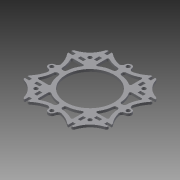
# Autodesk Inventor part: Plate2
Saved by Autodesk Inventor 2014 SP1 (Build 180222100, 222)
## iProperties
Created: 2014-07-27
Part Number: Plate2
Material: Generic
Document SubType Name: Modeling
Designer: Ryan
Density: 1 g/cm^3
Appearance: Default
Author: Ryan
Autodesk Inventor part; units mm, degrees
ref_plane "YZ Plane" through (0, 0, 0) normal (1, 0, 0) x (0, 1, 0)
ref_plane "XZ Plane" through (0, 0, 0) normal (0, 1, 0) x (-1, 0, 0)
ref_plane "XY Plane" through (0, 0, 0) normal (0, 0, 1) x (1, 0, 0)
sketch "Plate2" plane through (0, 0, 0) normal (0, 0, 1) x (1, 0, 0)
  arc A0 (128.4552, 70.0073) -> (126.9175, 69.5516) centre (128.2368, 67.9221) ccw
  arc A1 (95.9929, 69.5516) -> (94.4552, 70.0073) centre (94.6736, 67.9221) ccw
  arc A2 (85.5189, 60.9436) -> (90.0883, 68.5842) centre (72.6151, 73.8474) ccw
  arc A3 (92.0552, 69.9919) -> (90.0883, 68.5842) centre (91.9751, 68.0259) ccw
  arc A4 (132.8221, 68.5842) -> (137.3915, 60.9436) centre (150.2953, 73.8474) ccw
  arc A5 (132.8221, 68.5842) -> (130.8552, 69.9919) centre (130.9353, 68.0259) ccw
  circle A6 centre (111.4552, 35.0073) radius 20
  line L0 (94.4552, 70.0073) -> (94.4552, 66.3006)
  line L1 (92.0552, 69.9919) -> (92.0552, 66.3006)
  line L2 (92.0552, 66.3006) -> (94.4552, 66.3006)
  line L3 (130.8552, 69.9919) -> (130.8552, 66.3073)
  line L4 (128.4552, 70.0073) -> (128.4552, 66.3073)
  line L5 (128.4552, 66.3073) -> (130.8552, 66.3073)
  line L6 (96.8417, 55.1789) -> (96.8417, 63.4787)
  arc A7 (98.3161, 64.359) -> (108.0321, 61.6397) centre (109.2141, 84.5799) ccw
  arc A8 (98.3161, 64.359) -> (96.8417, 63.4787) centre (97.8417, 63.4787) ccw
  arc A9 (109.4549, 60.1414) -> (108.0321, 61.6397) centre (107.9549, 60.1417) ccw
  arc A10 (108.0698, 57.6324) -> (98.3885, 54.3416) centre (109.6496, 37.0981) ccw
  arc A11 (96.8417, 55.1789) -> (98.3885, 54.3416) centre (97.8417, 55.1789) ccw
  arc A12 (108.0698, 57.6324) -> (109.4548, 59.1277) centre (107.9548, 59.128) ccw
  line L7 (109.4548, 59.1277) -> (109.4549, 60.1414)
  line L8 (126.0687, 55.1789) -> (126.0687, 63.4787)
  arc A13 (114.8782, 61.6397) -> (124.5943, 64.359) centre (113.6962, 84.5799) ccw
  arc A14 (126.0687, 63.4787) -> (124.5943, 64.359) centre (125.0687, 63.4787) ccw
  arc A15 (114.8782, 61.6397) -> (113.4554, 60.1414) centre (114.9554, 60.1417) ccw
  arc A16 (124.5219, 54.3416) -> (114.8405, 57.6324) centre (113.2608, 37.0981) ccw
  arc A17 (124.5219, 54.3416) -> (126.0687, 55.1789) centre (125.0687, 55.1789) ccw
  arc A18 (113.4556, 59.1277) -> (114.8405, 57.6324) centre (114.9556, 59.128) ccw
  line L9 (113.4556, 59.1277) -> (113.4554, 60.1414)
  line L10 (131.6268, 49.6208) -> (139.9266, 49.6208)
  arc A19 (140.8069, 48.1464) -> (138.0875, 38.4304) centre (161.0277, 37.2484) ccw
  arc A20 (140.8069, 48.1464) -> (139.9266, 49.6208) centre (139.9266, 48.6208) ccw
  arc A21 (136.5893, 37.0076) -> (138.0875, 38.4304) centre (136.5895, 38.5076) ccw
  arc A22 (134.0802, 38.3927) -> (130.7895, 48.074) centre (113.5459, 36.8129) ccw
  arc A23 (131.6268, 49.6208) -> (130.7895, 48.074) centre (131.6268, 48.6208) ccw
  arc A24 (134.0802, 38.3927) -> (135.5756, 37.0077) centre (135.5758, 38.5077) ccw
  line L11 (135.5756, 37.0077) -> (136.5893, 37.0076)
  line L12 (91.2836, 49.6208) -> (82.9838, 49.6208)
  arc A25 (84.8228, 38.4304) -> (82.1035, 48.1464) centre (61.8827, 37.2484) ccw
  arc A26 (82.9838, 49.6208) -> (82.1035, 48.1464) centre (82.9838, 48.6208) ccw
  arc A27 (84.8228, 38.4304) -> (86.3211, 37.0076) centre (86.3208, 38.5076) ccw
  arc A28 (92.1209, 48.074) -> (88.8301, 38.3927) centre (109.3644, 36.8129) ccw
  arc A29 (92.1209, 48.074) -> (91.2836, 49.6208) centre (91.2836, 48.6208) ccw
  arc A30 (87.3348, 37.0077) -> (88.8301, 38.3927) centre (87.3345, 38.5077) ccw
  line L13 (87.3348, 37.0077) -> (86.3211, 37.0076)
  arc A31 (145.9995, 50.4696) -> (146.4552, 52.0073) centre (144.3699, 51.7889) ccw
  arc A32 (137.3915, 60.9436) -> (145.032, 56.3742) centre (150.2953, 73.8474) ccw
  arc A33 (146.4397, 54.4073) -> (145.032, 56.3742) centre (144.4737, 54.4874) ccw
  line L14 (146.4397, 54.4073) -> (142.7552, 54.4073)
  line L15 (146.4552, 52.0073) -> (142.7552, 52.0073)
  line L16 (142.7552, 52.0073) -> (142.7552, 54.4073)
  arc A34 (81.7248, 40.9245) -> (76.9109, 50.4696) centre (58.1218, 35.0073) ccw
  arc A35 (76.4552, 52.0073) -> (76.9109, 50.4696) centre (78.5404, 51.7889) ccw
  arc A36 (77.8783, 56.3742) -> (85.5189, 60.9436) centre (72.6151, 73.8474) ccw
  arc A37 (77.8783, 56.3742) -> (76.4706, 54.4073) centre (78.4366, 54.4874) ccw
  line L17 (76.4552, 52.0073) -> (80.1619, 52.0073)
  line L18 (76.4706, 54.4073) -> (80.1619, 54.4073)
  line L19 (80.1619, 54.4073) -> (80.1619, 52.0073)
  arc A38 (126.9175, 0.463) -> (128.4552, 0.0073) centre (128.2368, 2.0926) ccw
  arc A39 (94.4552, 0.0073) -> (95.9929, 0.463) centre (94.6736, 2.0926) ccw
  arc A40 (90.0883, 1.4305) -> (85.5189, 9.071) centre (72.6151, -3.8328) ccw
  arc A41 (90.0883, 1.4305) -> (92.0552, 0.0228) centre (91.9751, 1.9888) ccw
  arc A42 (137.3915, 9.071) -> (132.8221, 1.4305) centre (150.2953, -3.8328) ccw
  arc A43 (130.8552, 0.0228) -> (132.8221, 1.4305) centre (130.9353, 1.9888) ccw
  line L20 (94.4552, 0.0073) -> (94.4552, 3.7141)
  line L21 (92.0552, 0.0228) -> (92.0552, 3.7141)
  line L22 (92.0552, 3.7141) -> (94.4552, 3.7141)
  line L23 (130.8552, 0.0228) -> (130.8552, 3.7073)
  line L24 (128.4552, 0.0073) -> (128.4552, 3.7073)
  line L25 (128.4552, 3.7073) -> (130.8552, 3.7073)
  line L26 (96.8417, 14.8357) -> (96.8417, 6.5359)
  arc A44 (108.0321, 8.375) -> (98.3161, 5.6556) centre (109.2141, -14.5652) ccw
  arc A45 (96.8417, 6.5359) -> (98.3161, 5.6556) centre (97.8417, 6.5359) ccw
  arc A46 (108.0321, 8.375) -> (109.4549, 9.8732) centre (107.9549, 9.873) ccw
  arc A47 (98.3885, 15.673) -> (108.0698, 12.3823) centre (109.6496, 32.9166) ccw
  arc A48 (98.3885, 15.673) -> (96.8417, 14.8357) centre (97.8417, 14.8357) ccw
  arc A49 (109.4548, 10.8869) -> (108.0698, 12.3823) centre (107.9548, 10.8867) ccw
  line L27 (109.4548, 10.8869) -> (109.4549, 9.8732)
  line L28 (126.0687, 14.8357) -> (126.0687, 6.5359)
  arc A50 (124.5943, 5.6556) -> (114.8782, 8.375) centre (113.6962, -14.5652) ccw
  arc A51 (124.5943, 5.6556) -> (126.0687, 6.5359) centre (125.0687, 6.5359) ccw
  arc A52 (113.4554, 9.8732) -> (114.8782, 8.375) centre (114.9554, 9.873) ccw
  arc A53 (114.8405, 12.3823) -> (124.5219, 15.673) centre (113.2608, 32.9166) ccw
  arc A54 (126.0687, 14.8357) -> (124.5219, 15.673) centre (125.0687, 14.8357) ccw
  arc A55 (114.8405, 12.3823) -> (113.4556, 10.8869) centre (114.9556, 10.8867) ccw
  line L29 (113.4556, 10.8869) -> (113.4554, 9.8732)
  line L30 (131.6268, 20.3938) -> (139.9266, 20.3938)
  arc A56 (138.0875, 31.5843) -> (140.8069, 21.8682) centre (161.0277, 32.7663) ccw
  arc A57 (139.9266, 20.3938) -> (140.8069, 21.8682) centre (139.9266, 21.3938) ccw
  arc A58 (138.0875, 31.5843) -> (136.5893, 33.0071) centre (136.5895, 31.5071) ccw
  arc A59 (130.7895, 21.9406) -> (134.0802, 31.622) centre (113.5459, 33.2017) ccw
  arc A60 (130.7895, 21.9406) -> (131.6268, 20.3938) centre (131.6268, 21.3938) ccw
  arc A61 (135.5756, 33.0069) -> (134.0802, 31.622) centre (135.5758, 31.5069) ccw
  line L31 (135.5756, 33.0069) -> (136.5893, 33.0071)
  line L32 (91.2836, 20.3938) -> (82.9838, 20.3938)
  arc A62 (82.1035, 21.8682) -> (84.8228, 31.5843) centre (61.8827, 32.7663) ccw
  arc A63 (82.1035, 21.8682) -> (82.9838, 20.3938) centre (82.9838, 21.3938) ccw
  arc A64 (86.3211, 33.0071) -> (84.8228, 31.5843) centre (86.3208, 31.5071) ccw
  arc A65 (88.8301, 31.622) -> (92.1209, 21.9406) centre (109.3644, 33.2017) ccw
  arc A66 (91.2836, 20.3938) -> (92.1209, 21.9406) centre (91.2836, 21.3938) ccw
  arc A67 (88.8301, 31.622) -> (87.3348, 33.0069) centre (87.3345, 31.5069) ccw
  line L33 (87.3348, 33.0069) -> (86.3211, 33.0071)
  arc A68 (146.4552, 18.0073) -> (145.9995, 19.545) centre (144.3699, 18.2257) ccw
  arc A69 (145.032, 13.6404) -> (137.3915, 9.071) centre (150.2953, -3.8328) ccw
  arc A70 (145.032, 13.6404) -> (146.4397, 15.6073) centre (144.4737, 15.5272) ccw
  line L34 (146.4397, 15.6073) -> (142.7552, 15.6073)
  line L35 (146.4552, 18.0073) -> (142.7552, 18.0073)
  line L36 (142.7552, 18.0073) -> (142.7552, 15.6073)
  arc A71 (76.9109, 19.545) -> (81.7248, 29.0902) centre (58.1218, 35.0073) ccw
  arc A72 (76.9109, 19.545) -> (76.4552, 18.0073) centre (78.5404, 18.2257) ccw
  arc A73 (85.5189, 9.071) -> (77.8783, 13.6404) centre (72.6151, -3.8328) ccw
  arc A74 (76.4706, 15.6073) -> (77.8783, 13.6404) centre (78.4366, 15.5272) ccw
  line L37 (76.4552, 18.0073) -> (80.1619, 18.0073)
  line L38 (76.4706, 15.6073) -> (80.1619, 15.6073)
  line L39 (80.1619, 15.6073) -> (80.1619, 18.0073)
  circle A75 centre (79.6354, 35.0073) radius 1.6
  circle A76 centre (88.9552, 12.5073) radius 1.6
  circle A77 centre (88.9552, 57.5073) radius 1.6
  circle A78 centre (133.9552, 57.5073) radius 1.6
  circle A79 centre (133.9552, 12.5073) radius 1.6
  arc A80 (76.8156, 35.0073) -> (79.4575, 32.1931) centre (79.6354, 35.0073) ccw
  arc A81 (79.4575, 37.8215) -> (76.8156, 35.0073) centre (79.6354, 35.0073) ccw
  arc A82 (79.4575, 37.8215) -> (81.7248, 40.9245) centre (79.2998, 40.3165) ccw
  arc A83 (81.7248, 29.0902) -> (79.4575, 32.1931) centre (79.2998, 29.6981) ccw
  arc A84 (95.9929, 69.5516) -> (105.538, 64.7377) centre (111.4552, 88.3407) ccw
  arc A85 (117.3723, 64.7377) -> (126.9175, 69.5516) centre (111.4552, 88.3407) ccw
  arc A86 (114.2694, 67.005) -> (117.3723, 64.7377) centre (116.7644, 67.1627) ccw
  circle A87 centre (111.4552, 66.8271) radius 1.6
  arc A88 (114.2694, 67.005) -> (111.4552, 69.6469) centre (111.4552, 66.8271) ccw
  arc A89 (111.4552, 69.6469) -> (108.641, 67.005) centre (111.4552, 66.8271) ccw
  arc A90 (105.538, 64.7377) -> (108.641, 67.005) centre (106.146, 67.1627) ccw
  arc A91 (145.9995, 50.4696) -> (141.1856, 40.9245) centre (164.7885, 35.0073) ccw
  arc A92 (141.1856, 29.0902) -> (145.9995, 19.545) centre (164.7885, 35.0073) ccw
  arc A93 (143.4528, 32.1931) -> (141.1856, 29.0902) centre (143.6105, 29.6981) ccw
  circle A94 centre (143.275, 35.0073) radius 1.6
  arc A95 (143.4528, 32.1931) -> (146.0948, 35.0073) centre (143.275, 35.0073) ccw
  arc A96 (146.0948, 35.0073) -> (143.4528, 37.8215) centre (143.275, 35.0073) ccw
  arc A97 (141.1856, 40.9245) -> (143.4528, 37.8215) centre (143.6105, 40.3165) ccw
  arc A98 (105.538, 5.2769) -> (95.9929, 0.463) centre (111.4552, -18.326) ccw
  arc A99 (126.9175, 0.463) -> (117.3723, 5.2769) centre (111.4552, -18.326) ccw
  arc A100 (117.3723, 5.2769) -> (114.2694, 3.0097) centre (116.7644, 2.852) ccw
  circle A101 centre (111.4552, 3.1875) radius 1.6
  arc A102 (111.4552, 0.3677) -> (114.2694, 3.0097) centre (111.4552, 3.1875) ccw
  arc A103 (108.641, 3.0097) -> (111.4552, 0.3677) centre (111.4552, 3.1875) ccw
  arc A104 (108.641, 3.0097) -> (105.538, 5.2769) centre (106.146, 2.852) ccw
  line L40 (84.3552, 52.0073) -> (84.3552, 54.4073)
  line L41 (84.3552, 54.4073) -> (88.7552, 54.4073)
  line L42 (88.7552, 54.4073) -> (88.7552, 52.0073)
  line L43 (88.7552, 52.0073) -> (84.3552, 52.0073)
  line L44 (138.5552, 54.4073) -> (134.1552, 54.4073)
  line L45 (134.1552, 54.4073) -> (134.1552, 52.0072)
  line L46 (134.1552, 52.0072) -> (138.5552, 52.0073)
  line L47 (138.5552, 52.0073) -> (138.5552, 54.4073)
  line L48 (84.3552, 18.0073) -> (84.3552, 15.6073)
  line L49 (84.3552, 15.6073) -> (88.7552, 15.6073)
  line L50 (84.3552, 18.0073) -> (88.7552, 18.0073)
  line L51 (88.7552, 18.0073) -> (88.7552, 15.6073)
  line L52 (138.5552, 18.0073) -> (138.5552, 15.6073)
  line L53 (138.5552, 15.6073) -> (134.1552, 15.6073)
  line L54 (138.5552, 18.0073) -> (134.1552, 18.0073)
  line L55 (134.1552, 18.0073) -> (134.1552, 15.6073)
  line L56 (92.0552, 62.1073) -> (94.4552, 62.1073)
  line L57 (94.4552, 62.1073) -> (94.4552, 57.7073)
  line L58 (92.0552, 62.1073) -> (92.0552, 57.7073)
  line L59 (92.0552, 57.7073) -> (94.4552, 57.7073)
  line L60 (128.4552, 62.1073) -> (130.8552, 62.1073)
  line L61 (130.8552, 62.1073) -> (130.8552, 57.7073)
  line L62 (128.4552, 62.1073) -> (128.4552, 57.7073)
  line L63 (128.4552, 57.7073) -> (130.8552, 57.7073)
  line L64 (128.4552, 7.9073) -> (130.8552, 7.9073)
  line L65 (130.8552, 7.9073) -> (130.8552, 12.3073)
  line L66 (128.4552, 7.9073) -> (128.4552, 12.3073)
  line L67 (128.4552, 12.3073) -> (130.8552, 12.3073)
  line L68 (92.0552, 7.9073) -> (94.4552, 7.9073)
  line L69 (94.4552, 7.9073) -> (94.4552, 12.3073)
  line L70 (92.0552, 7.9073) -> (92.0552, 12.3073)
  line L71 (92.0552, 12.3073) -> (94.4552, 12.3073)
  point P0 (111.4553, 35.0073)
sketch "Sketch1" plane through (0, 0, 0) normal (0, 1, 0) x (-1, 0, 0)
  circle A0 centre (35.6381, 35.0073) radius 20
  circle A1 centre (67.4579, 35.0073) radius 1.6
  circle A2 centre (35.6381, 66.8271) radius 1.6
  circle A3 centre (13.1381, 57.5073) radius 1.6
  circle A4 centre (58.1381, 57.5073) radius 1.6
  circle A5 centre (3.8183, 35.0073) radius 1.6
  circle A6 centre (13.1381, 12.5073) radius 1.6
  circle A7 centre (35.6381, 3.1875) radius 1.6
  circle A8 centre (58.1381, 12.5073) radius 1.6
  line L0 (8.5381, 54.4073) -> (12.9381, 54.4073)
  line L1 (12.9381, 54.4073) -> (12.9381, 52.0073)
  line L2 (12.9381, 52.0073) -> (8.5381, 52.0073)
  line L3 (8.5381, 52.0073) -> (8.5381, 54.4073)
  line L4 (16.2381, 62.1073) -> (18.6381, 62.1073)
  line L5 (18.6381, 62.1073) -> (18.6381, 57.7073)
  line L6 (18.6381, 57.7073) -> (16.2381, 57.7073)
  line L7 (16.2381, 57.7073) -> (16.2381, 62.1073)
  line L8 (52.6381, 62.1073) -> (55.0381, 62.1073)
  line L9 (55.0381, 62.1073) -> (55.0381, 57.7073)
  line L10 (55.0381, 57.7073) -> (52.6381, 57.7073)
  line L11 (52.6381, 57.7073) -> (52.6381, 62.1073)
  line L12 (58.3381, 54.4073) -> (62.7381, 54.4073)
  line L13 (62.7381, 54.4073) -> (62.7381, 52.0073)
  line L14 (62.7381, 52.0073) -> (58.3381, 52.0073)
  line L15 (58.3381, 52.0073) -> (58.3381, 54.4073)
  line L16 (58.3381, 18.0073) -> (62.7381, 18.0073)
  line L17 (62.7381, 18.0073) -> (62.7381, 15.6073)
  line L18 (62.7381, 15.6073) -> (58.3381, 15.6073)
  line L19 (58.3381, 15.6073) -> (58.3381, 18.0073)
  line L20 (52.6381, 12.3073) -> (55.0381, 12.3073)
  line L21 (55.0381, 12.3073) -> (55.0381, 7.9073)
  line L22 (55.0381, 7.9073) -> (52.6381, 7.9073)
  line L23 (52.6381, 7.9073) -> (52.6381, 12.3073)
  line L24 (16.2381, 12.3073) -> (18.6381, 12.3073)
  line L25 (18.6381, 12.3073) -> (18.6381, 7.9073)
  line L26 (18.6381, 7.9073) -> (16.2381, 7.9073)
  line L27 (16.2381, 7.9073) -> (16.2381, 12.3073)
  line L28 (8.5381, 18.0073) -> (12.9381, 18.0073)
  line L29 (12.9381, 18.0073) -> (12.9381, 15.6073)
  line L30 (12.9381, 15.6073) -> (8.5381, 15.6073)
  line L31 (8.5381, 15.6073) -> (8.5381, 18.0073)
  arc A9 (14.2762, 1.4139) -> (2.0446, 13.6454) centre (-3.2021, -3.8328) ccw
  arc A10 (69.2315, 13.6454) -> (56.9999, 1.4139) centre (74.4782, -3.8328) ccw
  arc A11 (56.9999, 68.6008) -> (69.2315, 56.3692) centre (74.4782, 73.8474) ccw
  arc A12 (2.0446, 56.3692) -> (14.2762, 68.6008) centre (-3.2021, 73.8474) ccw
  arc A13 (57.0049, 68.5842) -> (55.0381, 69.9919) centre (55.1182, 68.0259) ccw
  arc A14 (52.6381, 70.0073) -> (51.0765, 69.532) centre (52.4197, 67.9221) ccw
  arc A15 (0.6535, 15.6073) -> (2.0612, 13.6404) centre (2.6195, 15.5272) ccw
  arc A16 (1.1134, 19.5689) -> (0.6381, 18.0073) centre (2.7233, 18.2257) ccw
  arc A17 (0.6381, 52.0073) -> (1.1134, 50.4458) centre (2.7233, 51.7889) ccw
  arc A18 (2.0612, 56.3742) -> (0.6535, 54.4073) centre (2.6195, 54.4874) ccw
  arc A19 (20.1996, 69.532) -> (18.6381, 70.0073) centre (18.8564, 67.9221) ccw
  arc A20 (17.5191, 66.3073) -> (17.5272, 66.3006) centre (18.8564, 67.9221) ccw
  arc A21 (16.2381, 69.9919) -> (14.2712, 68.5842) centre (16.158, 68.0259) ccw
  arc A22 (70.1627, 50.4458) -> (70.6381, 52.0073) centre (68.5528, 51.7889) ccw
  arc A23 (70.6226, 54.4073) -> (69.2149, 56.3742) centre (68.6566, 54.4874) ccw
  arc A24 (69.2149, 13.6404) -> (70.6226, 15.6073) centre (68.6566, 15.5272) ccw
  arc A25 (70.6381, 18.0073) -> (70.1627, 19.5689) centre (68.5528, 18.2257) ccw
  arc A26 (51.0765, 0.4827) -> (52.6381, 0.0073) centre (52.4197, 2.0926) ccw
  arc A27 (55.0381, 0.0228) -> (57.0049, 1.4305) centre (55.1182, 1.9888) ccw
  arc A28 (18.6381, 0.0073) -> (20.1996, 0.4827) centre (18.8564, 2.0926) ccw
  arc A29 (14.2712, 1.4305) -> (16.2381, 0.0228) centre (16.158, 1.9888) ccw
  arc A30 (5.9077, 29.0902) -> (3.6404, 32.1931) centre (3.4827, 29.6981) ccw
  arc A31 (3.6404, 37.8215) -> (5.9077, 40.9245) centre (3.4827, 40.3165) ccw
  arc A32 (29.7209, 64.7377) -> (32.8239, 67.005) centre (30.3288, 67.1627) ccw
  arc A33 (38.4522, 67.005) -> (41.5552, 64.7377) centre (40.9473, 67.1627) ccw
  arc A34 (38.4522, 67.005) -> (32.8239, 67.005) centre (35.6381, 66.8271) ccw
  arc A35 (3.6404, 37.8215) -> (3.6404, 32.1931) centre (3.8183, 35.0073) ccw
  arc A36 (67.6357, 32.1931) -> (67.6357, 37.8215) centre (67.4579, 35.0073) ccw
  arc A37 (65.3685, 40.9245) -> (67.6357, 37.8215) centre (67.7934, 40.3165) ccw
  arc A38 (67.6357, 32.1931) -> (65.3685, 29.0902) centre (67.7934, 29.6981) ccw
  arc A39 (41.5552, 5.2769) -> (38.4522, 3.0097) centre (40.9473, 2.852) ccw
  arc A40 (32.8239, 3.0097) -> (38.4522, 3.0097) centre (35.6381, 3.1875) ccw
  arc A41 (32.8239, 3.0097) -> (29.7209, 5.2769) centre (30.3288, 2.852) ccw
  arc A42 (1.0938, 19.545) -> (5.9077, 29.0902) centre (-17.6953, 35.0073) ccw
  arc A43 (5.9077, 40.9245) -> (1.0938, 50.4696) centre (-17.6953, 35.0073) ccw
  arc A44 (65.3685, 29.0902) -> (70.1824, 19.545) centre (88.9714, 35.0073) ccw
  arc A45 (70.1824, 50.4696) -> (65.3685, 40.9245) centre (88.9714, 35.0073) ccw
  arc A46 (20.1757, 69.5516) -> (29.7209, 64.7377) centre (35.6381, 88.3407) ccw
  arc A47 (41.5552, 64.7377) -> (51.1004, 69.5516) centre (35.6381, 88.3407) ccw
  arc A48 (29.7209, 5.2769) -> (20.1757, 0.463) centre (35.6381, -18.326) ccw
  arc A49 (51.1004, 0.463) -> (41.5552, 5.2769) centre (35.6381, -18.326) ccw
  line L32 (0.6381, 18.0073) -> (4.3448, 18.0073)
  line L33 (4.3448, 18.0073) -> (4.3448, 15.6073)
  line L34 (4.3448, 15.6073) -> (0.6535, 15.6073)
  line L35 (0.6381, 52.0073) -> (4.3448, 52.0073)
  line L36 (4.3448, 52.0073) -> (4.3448, 54.4073)
  line L37 (4.3448, 54.4073) -> (0.6535, 54.4073)
  line L38 (16.2381, 69.9919) -> (16.2381, 66.3006)
  line L39 (16.2381, 66.3006) -> (18.6381, 66.3006)
  line L40 (18.6381, 66.3006) -> (18.6381, 70.0073)
  line L41 (52.6381, 70.0073) -> (52.6381, 66.3073)
  line L42 (52.6381, 66.3073) -> (55.0381, 66.3073)
  line L43 (55.0381, 66.3073) -> (55.0381, 69.9919)
  line L44 (70.6226, 54.4073) -> (66.9381, 54.4073)
  line L45 (66.9381, 54.4073) -> (66.9381, 52.0073)
  line L46 (66.9381, 52.0073) -> (70.6381, 52.0073)
  line L47 (70.6226, 15.6073) -> (66.9381, 15.6073)
  line L48 (66.9381, 15.6073) -> (66.9381, 18.0073)
  line L49 (66.9381, 18.0073) -> (70.6381, 18.0073)
  line L50 (55.0381, 0.0228) -> (55.0381, 3.7073)
  line L51 (55.0381, 3.7073) -> (52.6381, 3.7073)
  line L52 (52.6381, 3.7073) -> (52.6381, 0.0073)
  line L53 (18.6381, 0.0073) -> (18.6381, 3.7141)
  line L54 (18.6381, 3.7141) -> (16.2381, 3.7141)
  line L55 (16.2381, 3.7141) -> (16.2381, 0.0228)
  arc A50 (6.2863, 21.8682) -> (7.1666, 20.3938) centre (7.1666, 21.3938) ccw
  arc A51 (15.4665, 20.3938) -> (16.3037, 21.9406) centre (15.4665, 21.3938) ccw
  arc A52 (13.013, 31.622) -> (11.5177, 33.0069) centre (11.5174, 31.5069) ccw
  arc A53 (10.504, 33.0071) -> (9.0057, 31.5843) centre (10.5037, 31.5071) ccw
  arc A54 (9.0057, 38.4304) -> (10.504, 37.0076) centre (10.5037, 38.5076) ccw
  arc A55 (7.1666, 49.6208) -> (6.2863, 48.1464) centre (7.1666, 48.6208) ccw
  arc A56 (16.3037, 48.074) -> (15.4665, 49.6208) centre (15.4665, 48.6208) ccw
  arc A57 (21.0245, 55.1789) -> (22.5713, 54.3416) centre (22.0245, 55.1789) ccw
  arc A58 (22.499, 64.359) -> (21.0245, 63.4787) centre (22.0245, 63.4787) ccw
  arc A59 (33.6378, 60.1414) -> (32.215, 61.6397) centre (32.1378, 60.1417) ccw
  arc A60 (32.2527, 57.6324) -> (33.6376, 59.1277) centre (32.1376, 59.128) ccw
  arc A61 (37.6385, 59.1277) -> (39.0234, 57.6324) centre (39.1385, 59.128) ccw
  arc A62 (39.0611, 61.6397) -> (37.6383, 60.1414) centre (39.1383, 60.1417) ccw
  arc A63 (50.2516, 63.4787) -> (48.7771, 64.359) centre (49.2516, 63.4787) ccw
  arc A64 (48.7048, 54.3416) -> (50.2516, 55.1789) centre (49.2516, 55.1789) ccw
  arc A65 (55.8096, 49.6208) -> (54.9724, 48.074) centre (55.8096, 48.6208) ccw
  arc A66 (64.9898, 48.1464) -> (64.1095, 49.6208) centre (64.1095, 48.6208) ccw
  arc A67 (60.7722, 37.0076) -> (62.2704, 38.4304) centre (60.7724, 38.5076) ccw
  arc A68 (58.2631, 38.3927) -> (59.7584, 37.0077) centre (59.7587, 38.5077) ccw
  arc A69 (59.7584, 33.0069) -> (58.2631, 31.622) centre (59.7587, 31.5069) ccw
  arc A70 (62.2704, 31.5843) -> (60.7722, 33.0071) centre (60.7724, 31.5071) ccw
  arc A71 (54.9724, 21.9406) -> (55.8096, 20.3938) centre (55.8096, 21.3938) ccw
  arc A72 (64.1095, 20.3938) -> (64.9898, 21.8682) centre (64.1095, 21.3938) ccw
  arc A73 (39.0234, 12.3823) -> (37.6385, 10.8869) centre (39.1385, 10.8867) ccw
  arc A74 (37.6383, 9.8732) -> (39.0611, 8.375) centre (39.1383, 9.873) ccw
  arc A75 (50.2516, 14.8357) -> (48.7048, 15.673) centre (49.2516, 14.8357) ccw
  arc A76 (48.7771, 5.6556) -> (50.2516, 6.5359) centre (49.2516, 6.5359) ccw
  arc A77 (21.0245, 6.5359) -> (22.499, 5.6556) centre (22.0245, 6.5359) ccw
  arc A78 (22.5713, 15.673) -> (21.0245, 14.8357) centre (22.0245, 14.8357) ccw
  arc A79 (33.6376, 10.8869) -> (32.2527, 12.3823) centre (32.1376, 10.8867) ccw
  arc A80 (32.215, 8.375) -> (33.6378, 9.8732) centre (32.1378, 9.873) ccw
  line L56 (21.0245, 14.8357) -> (21.0245, 6.5359)
  line L57 (50.2516, 6.5359) -> (50.2516, 14.8357)
  line L58 (7.1666, 20.3938) -> (15.4665, 20.3938)
  line L59 (7.1666, 49.6208) -> (15.4665, 49.6208)
  line L60 (21.0245, 55.1789) -> (21.0245, 63.4787)
  line L61 (50.2516, 63.4787) -> (50.2516, 55.1789)
  line L62 (55.8096, 49.6208) -> (64.1095, 49.6208)
  line L63 (55.8096, 20.3938) -> (64.1095, 20.3938)
  arc A81 (11.5177, 37.0077) -> (13.013, 38.3927) centre (11.5174, 38.5077) ccw
  line L64 (10.504, 37.0076) -> (11.5177, 37.0077)
  line L65 (10.504, 33.0071) -> (11.5177, 33.0069)
  line L66 (33.6376, 10.8869) -> (33.6378, 9.8732)
  line L67 (37.6383, 9.8732) -> (37.6385, 10.8869)
  line L68 (59.7584, 37.0077) -> (60.7722, 37.0076)
  line L69 (59.7584, 33.0069) -> (60.7722, 33.0071)
  line L70 (33.6378, 60.1414) -> (33.6376, 59.1277)
  line L71 (37.6383, 60.0997) -> (37.6385, 59.1277)
  arc A82 (32.215, 8.375) -> (22.499, 5.6556) centre (33.397, -14.5652) ccw
  arc A83 (48.7771, 5.6556) -> (39.0611, 8.375) centre (37.8791, -14.5652) ccw
  arc A84 (6.2863, 21.8682) -> (9.0057, 31.5843) centre (-13.9345, 32.7663) ccw
  arc A85 (9.0057, 38.4304) -> (6.2863, 48.1464) centre (-13.9345, 37.2484) ccw
  arc A86 (22.499, 64.359) -> (32.215, 61.6397) centre (33.397, 84.5799) ccw
  arc A87 (39.0611, 61.6397) -> (48.7771, 64.359) centre (37.8791, 84.5799) ccw
  arc A88 (62.2704, 31.5843) -> (64.9898, 21.8682) centre (85.2106, 32.7663) ccw
  arc A89 (64.9898, 48.1464) -> (62.2704, 38.4304) centre (85.2106, 37.2484) ccw
  arc A90 (22.5713, 15.673) -> (32.2527, 12.3823) centre (33.8324, 32.9166) ccw
  arc A91 (39.0234, 12.3823) -> (48.7048, 15.673) centre (37.4437, 32.9166) ccw
  arc A92 (13.013, 31.622) -> (16.3037, 21.9406) centre (33.5473, 33.2017) ccw
  arc A93 (16.3037, 48.074) -> (13.013, 38.3927) centre (33.5473, 36.8129) ccw
  arc A94 (32.2527, 57.6324) -> (22.5713, 54.3416) centre (33.8324, 37.0981) ccw
  arc A95 (48.7048, 54.3416) -> (39.0234, 57.6324) centre (37.4437, 37.0981) ccw
  arc A96 (58.2631, 38.3927) -> (54.9724, 48.074) centre (37.7288, 36.8129) ccw
  arc A97 (54.9724, 21.9406) -> (58.2631, 31.622) centre (37.7288, 33.2017) ccw
  arc A98 (3.6404, 37.8215) -> (3.6404, 32.1931) centre (3.8183, 35.0073) ccw
  arc A99 (3.6404, 37.8215) -> (5.9077, 40.9245) centre (3.4827, 40.3165) ccw
  arc A100 (5.9077, 40.9245) -> (1.0938, 50.4696) centre (-17.6953, 35.0073) ccw
  arc A101 (0.6381, 52.0073) -> (1.0938, 50.4696) centre (2.7233, 51.7889) ccw
  line L72 (0.6381, 52.0073) -> (4.3448, 52.0073)
  line L73 (4.3448, 52.0073) -> (4.3448, 54.4073)
  line L74 (4.3448, 54.4073) -> (0.6535, 54.4073)
  arc A102 (2.0612, 56.3742) -> (0.6535, 54.4073) centre (2.6195, 54.4874) ccw
  arc A103 (2.0612, 56.3742) -> (14.2712, 68.5842) centre (-3.2021, 73.8474) ccw
  arc A104 (16.2381, 69.9919) -> (14.2712, 68.5842) centre (16.158, 68.0259) ccw
  arc A105 (20.1996, 69.532) -> (18.6381, 70.0073) centre (18.8564, 67.9221) ccw
  arc A106 (20.1996, 69.532) -> (29.7209, 64.7377) centre (35.6381, 88.3407) ccw
  arc A107 (41.5552, 64.7377) -> (51.0765, 69.532) centre (35.6381, 88.3407) ccw
  arc A108 (52.6381, 70.0073) -> (51.0765, 69.532) centre (52.4197, 67.9221) ccw
  arc A109 (57.0049, 68.5842) -> (55.0381, 69.9919) centre (55.1182, 68.0259) ccw
  arc A110 (57.0049, 68.5842) -> (69.2149, 56.3742) centre (74.3462, 73.7154) ccw
  arc A111 (70.6226, 54.4073) -> (69.2149, 56.3742) centre (68.6566, 54.4874) ccw
  arc A112 (70.1627, 50.4458) -> (70.6381, 52.0073) centre (68.5528, 51.7889) ccw
  arc A113 (65.3685, 40.9245) -> (67.6357, 37.8215) centre (67.7934, 40.3165) ccw
  arc A114 (67.6357, 32.1931) -> (65.3685, 29.0902) centre (67.7934, 29.6981) ccw
  arc A115 (70.6381, 18.0073) -> (70.1627, 19.5689) centre (68.5528, 18.2257) ccw
  arc A116 (69.2149, 13.6404) -> (70.6226, 15.6073) centre (68.6566, 15.5272) ccw
  arc A117 (69.2149, 13.6404) -> (57.0049, 1.4305) centre (74.4782, -3.8328) ccw
  arc A118 (55.0381, 0.0228) -> (57.0049, 1.4305) centre (55.1182, 1.9888) ccw
  arc A119 (51.0765, 0.4827) -> (52.6381, 0.0073) centre (52.4197, 2.0926) ccw
  arc A120 (51.0765, 0.4827) -> (41.5552, 5.2769) centre (35.6381, -18.326) ccw
  arc A121 (29.7209, 5.2769) -> (20.1996, 0.4827) centre (35.6381, -18.326) ccw
  arc A122 (18.6381, 0.0073) -> (20.1996, 0.4827) centre (18.8564, 2.0926) ccw
  arc A123 (14.2712, 1.4305) -> (16.2381, 0.0228) centre (16.158, 1.9888) ccw
  arc A124 (14.2712, 1.4305) -> (2.0612, 13.6404) centre (-3.2021, -3.8328) ccw
  arc A125 (0.6535, 15.6073) -> (2.0612, 13.6404) centre (2.6195, 15.5272) ccw
  arc A126 (1.1134, 19.5689) -> (0.6381, 18.0073) centre (2.7233, 18.2257) ccw
  arc A127 (1.1134, 19.5689) -> (5.9077, 29.0902) centre (-17.6953, 35.0073) ccw
  arc A128 (3.6404, 37.8215) -> (5.9077, 40.9245) centre (3.4827, 40.3165) ccw
  arc A129 (5.9077, 40.9245) -> (1.0938, 50.4696) centre (-17.6953, 35.0073) ccw
  arc A130 (0.6381, 52.0073) -> (1.0938, 50.4696) centre (2.7233, 51.7889) ccw
  arc A131 (48.7048, 54.3416) -> (39.0234, 57.6324) centre (37.4437, 37.0981) ccw
  arc A132 (48.7048, 54.3416) -> (50.2516, 55.1789) centre (49.2516, 55.1789) ccw
  arc A133 (50.2516, 63.4787) -> (48.7771, 64.359) centre (49.2516, 63.4787) ccw
  arc A134 (39.0611, 61.6397) -> (48.7771, 64.359) centre (37.8791, 84.5799) ccw
  arc A135 (39.0611, 61.6397) -> (37.6383, 60.0997) centre (39.1388, 60.1407) ccw
  arc A136 (48.7048, 54.3416) -> (39.0234, 57.6324) centre (37.4437, 37.0981) ccw
  arc A137 (37.6385, 59.1277) -> (39.0234, 57.6324) centre (39.1385, 59.128) ccw
  line L75 (37.6385, 59.1277) -> (37.6383, 60.0997)
  line L76 (50.2516, 55.1789) -> (50.2516, 63.4787)
  arc A138 (52.6381, 70.0073) -> (51.1004, 69.5516) centre (52.4197, 67.9221) ccw
  arc A139 (20.1757, 69.5516) -> (18.6381, 70.0073) centre (18.8564, 67.9221) ccw
  arc A140 (9.7017, 60.9436) -> (14.2712, 68.5842) centre (-3.2021, 73.8474) ccw
  arc A141 (16.2381, 69.9919) -> (14.2712, 68.5842) centre (16.158, 68.0259) ccw
  arc A142 (57.0049, 68.5842) -> (61.5744, 60.9436) centre (74.4782, 73.8474) ccw
  arc A143 (57.0049, 68.5842) -> (55.0381, 69.9919) centre (55.1182, 68.0259) ccw
  circle A144 centre (35.6381, 35.0073) radius 20
  line L77 (18.6381, 70.0073) -> (18.6381, 66.3006)
  line L78 (16.2381, 69.9919) -> (16.2381, 66.3006)
  line L79 (16.2381, 66.3006) -> (18.6381, 66.3006)
  line L80 (55.0381, 69.9919) -> (55.0381, 66.3073)
  line L81 (52.6381, 70.0073) -> (52.6381, 66.3073)
  line L82 (52.6381, 66.3073) -> (55.0381, 66.3073)
  line L83 (21.0245, 55.1789) -> (21.0245, 63.4787)
  arc A145 (22.499, 64.359) -> (32.215, 61.6397) centre (33.397, 84.5799) ccw
  arc A146 (22.499, 64.359) -> (21.0245, 63.4787) centre (22.0245, 63.4787) ccw
  arc A147 (33.6378, 60.1414) -> (32.215, 61.6397) centre (32.1378, 60.1417) ccw
  arc A148 (32.2527, 57.6324) -> (22.5713, 54.3416) centre (33.8324, 37.0981) ccw
  arc A149 (21.0245, 55.1789) -> (22.5713, 54.3416) centre (22.0245, 55.1789) ccw
  arc A150 (32.2527, 57.6324) -> (33.6376, 59.1277) centre (32.1376, 59.128) ccw
  line L84 (33.6376, 59.1277) -> (33.6378, 60.1414)
  line L85 (50.2516, 55.1789) -> (50.2516, 63.4787)
  arc A151 (39.0611, 61.6397) -> (48.7771, 64.359) centre (37.8791, 84.5799) ccw
  arc A152 (50.2516, 63.4787) -> (48.7771, 64.359) centre (49.2516, 63.4787) ccw
  arc A153 (39.0611, 61.6397) -> (37.6383, 60.1414) centre (39.1383, 60.1417) ccw
  arc A154 (48.7048, 54.3416) -> (39.0234, 57.6324) centre (37.4437, 37.0981) ccw
  arc A155 (48.7048, 54.3416) -> (50.2516, 55.1789) centre (49.2516, 55.1789) ccw
  arc A156 (37.6385, 59.1277) -> (39.0234, 57.6324) centre (39.1385, 59.128) ccw
  line L86 (37.6385, 59.1277) -> (37.6383, 60.1414)
  line L87 (55.8096, 49.6208) -> (64.1095, 49.6208)
  arc A157 (64.9898, 48.1464) -> (62.2704, 38.4304) centre (85.2106, 37.2484) ccw
  arc A158 (64.9898, 48.1464) -> (64.1095, 49.6208) centre (64.1095, 48.6208) ccw
  arc A159 (60.7722, 37.0076) -> (62.2704, 38.4304) centre (60.7724, 38.5076) ccw
  arc A160 (58.2631, 38.3927) -> (54.9724, 48.074) centre (37.7288, 36.8129) ccw
  arc A161 (55.8096, 49.6208) -> (54.9724, 48.074) centre (55.8096, 48.6208) ccw
  arc A162 (58.2631, 38.3927) -> (59.7584, 37.0077) centre (59.7587, 38.5077) ccw
  line L88 (59.7584, 37.0077) -> (60.7722, 37.0076)
  line L89 (15.4665, 49.6208) -> (7.1666, 49.6208)
  arc A163 (9.0057, 38.4304) -> (6.2863, 48.1464) centre (-13.9345, 37.2484) ccw
  arc A164 (7.1666, 49.6208) -> (6.2863, 48.1464) centre (7.1666, 48.6208) ccw
  arc A165 (9.0057, 38.4304) -> (10.504, 37.0076) centre (10.5037, 38.5076) ccw
  arc A166 (16.3037, 48.074) -> (13.013, 38.3927) centre (33.5473, 36.8129) ccw
  arc A167 (16.3037, 48.074) -> (15.4665, 49.6208) centre (15.4665, 48.6208) ccw
  arc A168 (11.5177, 37.0077) -> (13.013, 38.3927) centre (11.5174, 38.5077) ccw
  line L90 (11.5177, 37.0077) -> (10.504, 37.0076)
  arc A169 (70.1824, 50.4696) -> (70.6381, 52.0073) centre (68.5528, 51.7889) ccw
  arc A170 (61.5744, 60.9436) -> (69.2149, 56.3742) centre (74.4782, 73.8474) ccw
  arc A171 (70.6226, 54.4073) -> (69.2149, 56.3742) centre (68.6566, 54.4874) ccw
  line L91 (70.6226, 54.4073) -> (66.9381, 54.4073)
  line L92 (70.6381, 52.0073) -> (66.9381, 52.0073)
  line L93 (66.9381, 52.0073) -> (66.9381, 54.4073)
  arc A172 (5.9077, 40.9245) -> (1.0938, 50.4696) centre (-17.6953, 35.0073) ccw
  arc A173 (0.6381, 52.0073) -> (1.0938, 50.4696) centre (2.7233, 51.7889) ccw
  arc A174 (2.0612, 56.3742) -> (9.7017, 60.9436) centre (-3.2021, 73.8474) ccw
  arc A175 (2.0612, 56.3742) -> (0.6535, 54.4073) centre (2.6195, 54.4874) ccw
  line L94 (0.6381, 52.0073) -> (4.3448, 52.0073)
  line L95 (0.6535, 54.4073) -> (4.3448, 54.4073)
  line L96 (4.3448, 54.4073) -> (4.3448, 52.0073)
  arc A176 (51.1004, 0.463) -> (52.6381, 0.0073) centre (52.4197, 2.0926) ccw
  arc A177 (18.6381, 0.0073) -> (20.1757, 0.463) centre (18.8564, 2.0926) ccw
  arc A178 (14.2712, 1.4305) -> (9.7017, 9.071) centre (-3.2021, -3.8328) ccw
  arc A179 (14.2712, 1.4305) -> (16.2381, 0.0228) centre (16.158, 1.9888) ccw
  arc A180 (61.5744, 9.071) -> (57.0049, 1.4305) centre (74.4782, -3.8328) ccw
  arc A181 (55.0381, 0.0228) -> (57.0049, 1.4305) centre (55.1182, 1.9888) ccw
  line L97 (18.6381, 0.0073) -> (18.6381, 3.7141)
  line L98 (16.2381, 0.0228) -> (16.2381, 3.7141)
  line L99 (16.2381, 3.7141) -> (18.6381, 3.7141)
  line L100 (55.0381, 0.0228) -> (55.0381, 3.7073)
  line L101 (52.6381, 0.0073) -> (52.6381, 3.7073)
  line L102 (52.6381, 3.7073) -> (55.0381, 3.7073)
  line L103 (21.0245, 14.8357) -> (21.0245, 6.5359)
  arc A182 (32.215, 8.375) -> (22.499, 5.6556) centre (33.397, -14.5652) ccw
  arc A183 (21.0245, 6.5359) -> (22.499, 5.6556) centre (22.0245, 6.5359) ccw
  arc A184 (32.215, 8.375) -> (33.6378, 9.8732) centre (32.1378, 9.873) ccw
  arc A185 (22.5713, 15.673) -> (32.2527, 12.3823) centre (33.8324, 32.9166) ccw
  arc A186 (22.5713, 15.673) -> (21.0245, 14.8357) centre (22.0245, 14.8357) ccw
  arc A187 (33.6376, 10.8869) -> (32.2527, 12.3823) centre (32.1376, 10.8867) ccw
  line L104 (33.6376, 10.8869) -> (33.6378, 9.8732)
  line L105 (50.2516, 14.8357) -> (50.2516, 6.5359)
  arc A188 (48.7771, 5.6556) -> (39.0611, 8.375) centre (37.8791, -14.5652) ccw
  arc A189 (48.7771, 5.6556) -> (50.2516, 6.5359) centre (49.2516, 6.5359) ccw
  arc A190 (37.6383, 9.8732) -> (39.0611, 8.375) centre (39.1383, 9.873) ccw
  arc A191 (39.0234, 12.3823) -> (48.7048, 15.673) centre (37.4437, 32.9166) ccw
  arc A192 (50.2516, 14.8357) -> (48.7048, 15.673) centre (49.2516, 14.8357) ccw
  arc A193 (39.0234, 12.3823) -> (37.6385, 10.8869) centre (39.1385, 10.8867) ccw
  line L106 (37.6385, 10.8869) -> (37.6383, 9.8732)
  line L107 (55.8096, 20.3938) -> (64.1095, 20.3938)
  arc A194 (62.2704, 31.5843) -> (64.9898, 21.8682) centre (85.2106, 32.7663) ccw
  arc A195 (64.1095, 20.3938) -> (64.9898, 21.8682) centre (64.1095, 21.3938) ccw
  arc A196 (62.2704, 31.5843) -> (60.7722, 33.0071) centre (60.7724, 31.5071) ccw
  arc A197 (54.9724, 21.9406) -> (58.2631, 31.622) centre (37.7288, 33.2017) ccw
  arc A198 (54.9724, 21.9406) -> (55.8096, 20.3938) centre (55.8096, 21.3938) ccw
  arc A199 (59.7584, 33.0069) -> (58.2631, 31.622) centre (59.7587, 31.5069) ccw
  line L108 (59.7584, 33.0069) -> (60.7722, 33.0071)
  line L109 (15.4665, 20.3938) -> (7.1666, 20.3938)
  arc A200 (6.2863, 21.8682) -> (9.0057, 31.5843) centre (-13.9345, 32.7663) ccw
  arc A201 (6.2863, 21.8682) -> (7.1666, 20.3938) centre (7.1666, 21.3938) ccw
  arc A202 (10.504, 33.0071) -> (9.0057, 31.5843) centre (10.5037, 31.5071) ccw
  arc A203 (13.013, 31.622) -> (16.3037, 21.9406) centre (33.5473, 33.2017) ccw
  arc A204 (15.4665, 20.3938) -> (16.3037, 21.9406) centre (15.4665, 21.3938) ccw
  arc A205 (13.013, 31.622) -> (11.5177, 33.0069) centre (11.5174, 31.5069) ccw
  line L110 (11.5177, 33.0069) -> (10.504, 33.0071)
  arc A206 (70.6381, 18.0073) -> (70.1824, 19.545) centre (68.5528, 18.2257) ccw
  arc A207 (69.2149, 13.6404) -> (61.5744, 9.071) centre (74.4782, -3.8328) ccw
  arc A208 (69.2149, 13.6404) -> (70.6226, 15.6073) centre (68.6566, 15.5272) ccw
  line L111 (70.6226, 15.6073) -> (66.9381, 15.6073)
  line L112 (70.6381, 18.0073) -> (66.9381, 18.0073)
  line L113 (66.9381, 18.0073) -> (66.9381, 15.6073)
  arc A209 (1.0938, 19.545) -> (5.9077, 29.0902) centre (-17.6953, 35.0073) ccw
  arc A210 (1.0938, 19.545) -> (0.6381, 18.0073) centre (2.7233, 18.2257) ccw
  arc A211 (9.7017, 9.071) -> (2.0612, 13.6404) centre (-3.2021, -3.8328) ccw
  arc A212 (0.6535, 15.6073) -> (2.0612, 13.6404) centre (2.6195, 15.5272) ccw
  line L114 (0.6381, 18.0073) -> (4.3448, 18.0073)
  line L115 (0.6535, 15.6073) -> (4.3448, 15.6073)
  line L116 (4.3448, 15.6073) -> (4.3448, 18.0073)
  circle A213 centre (3.8183, 35.0073) radius 1.6
  circle A214 centre (13.1381, 12.5073) radius 1.6
  circle A215 centre (13.1381, 57.5073) radius 1.6
  circle A216 centre (58.1381, 57.5073) radius 1.6
  circle A217 centre (58.1381, 12.5073) radius 1.6
  arc A218 (0.9984, 35.0073) -> (3.6404, 32.1931) centre (3.8183, 35.0073) ccw
  arc A219 (3.6404, 37.8215) -> (0.9984, 35.0073) centre (3.8183, 35.0073) ccw
  arc A220 (3.6404, 37.8215) -> (5.9077, 40.9245) centre (3.4827, 40.3165) ccw
  arc A221 (5.9077, 29.0902) -> (3.6404, 32.1931) centre (3.4827, 29.6981) ccw
  arc A222 (20.1757, 69.5516) -> (29.7209, 64.7377) centre (35.6381, 88.3407) ccw
  arc A223 (41.5552, 64.7377) -> (51.1004, 69.5516) centre (35.6381, 88.3407) ccw
  arc A224 (38.4522, 67.005) -> (41.5552, 64.7377) centre (40.9473, 67.1627) ccw
  circle A225 centre (35.6381, 66.8271) radius 1.6
  arc A226 (38.4522, 67.005) -> (35.6381, 69.6469) centre (35.6381, 66.8271) ccw
  arc A227 (35.6381, 69.6469) -> (32.8239, 67.005) centre (35.6381, 66.8271) ccw
  arc A228 (29.7209, 64.7377) -> (32.8239, 67.005) centre (30.3288, 67.1627) ccw
  arc A229 (70.1824, 50.4696) -> (65.3685, 40.9245) centre (88.9714, 35.0073) ccw
  arc A230 (65.3685, 29.0902) -> (70.1824, 19.545) centre (88.9714, 35.0073) ccw
  arc A231 (67.6357, 32.1931) -> (65.3685, 29.0902) centre (67.7934, 29.6981) ccw
  circle A232 centre (67.4579, 35.0073) radius 1.6
  arc A233 (67.6357, 32.1931) -> (70.2777, 35.0073) centre (67.4579, 35.0073) ccw
  arc A234 (70.2777, 35.0073) -> (67.6357, 37.8215) centre (67.4579, 35.0073) ccw
  arc A235 (65.3685, 40.9245) -> (67.6357, 37.8215) centre (67.7934, 40.3165) ccw
  arc A236 (29.7209, 5.2769) -> (20.1757, 0.463) centre (35.6381, -18.326) ccw
  arc A237 (51.1004, 0.463) -> (41.5552, 5.2769) centre (35.6381, -18.326) ccw
  arc A238 (41.5552, 5.2769) -> (38.4522, 3.0097) centre (40.9473, 2.852) ccw
  circle A239 centre (35.6381, 3.1875) radius 1.6
  arc A240 (35.6381, 0.3677) -> (38.4522, 3.0097) centre (35.6381, 3.1875) ccw
  arc A241 (32.8239, 3.0097) -> (35.6381, 0.3677) centre (35.6381, 3.1875) ccw
  arc A242 (32.8239, 3.0097) -> (29.7209, 5.2769) centre (30.3288, 2.852) ccw
  line L117 (8.5381, 52.0073) -> (8.5381, 54.4073)
  line L118 (8.5381, 54.4073) -> (12.9381, 54.4073)
  line L119 (12.9381, 54.4073) -> (12.9381, 52.0073)
  line L120 (12.9381, 52.0073) -> (8.5381, 52.0073)
  line L121 (62.7381, 54.4073) -> (58.3381, 54.4073)
  line L122 (58.3381, 54.4073) -> (58.3381, 52.0072)
  line L123 (58.3381, 52.0072) -> (62.7381, 52.0073)
  line L124 (62.7381, 52.0073) -> (62.7381, 54.4073)
  line L125 (8.5381, 18.0073) -> (8.5381, 15.6073)
  line L126 (8.5381, 15.6073) -> (12.9381, 15.6073)
  line L127 (8.5381, 18.0073) -> (12.9381, 18.0073)
  line L128 (12.9381, 18.0073) -> (12.9381, 15.6073)
  line L129 (62.7381, 18.0073) -> (62.7381, 15.6073)
  line L130 (62.7381, 15.6073) -> (58.3381, 15.6073)
  line L131 (62.7381, 18.0073) -> (58.3381, 18.0073)
  line L132 (58.3381, 18.0073) -> (58.3381, 15.6073)
  line L133 (16.2381, 62.1073) -> (18.6381, 62.1073)
  line L134 (18.6381, 62.1073) -> (18.6381, 57.7073)
  line L135 (16.2381, 62.1073) -> (16.2381, 57.7073)
  line L136 (16.2381, 57.7073) -> (18.6381, 57.7073)
  line L137 (52.6381, 62.1073) -> (55.0381, 62.1073)
  line L138 (55.0381, 62.1073) -> (55.0381, 57.7073)
  line L139 (52.6381, 62.1073) -> (52.6381, 57.7073)
  line L140 (52.6381, 57.7073) -> (55.0381, 57.7073)
  line L141 (52.6381, 7.9073) -> (55.0381, 7.9073)
  line L142 (55.0381, 7.9073) -> (55.0381, 12.3073)
  line L143 (52.6381, 7.9073) -> (52.6381, 12.3073)
  line L144 (52.6381, 12.3073) -> (55.0381, 12.3073)
  line L145 (16.2381, 7.9073) -> (18.6381, 7.9073)
  line L146 (18.6381, 7.9073) -> (18.6381, 12.3073)
  line L147 (16.2381, 7.9073) -> (16.2381, 12.3073)
  line L148 (16.2381, 12.3073) -> (18.6381, 12.3073)
  point P0 (0, 0)
  constraints: 270 point on circle, 154 end point, 138 centre point, 31 tangent, 29 horizontal, 23 vertical, 17 parallel, 11 concentric, 11 perpendicular, 4 coincident, 3 collinear, 2 equal length, 291 other
extrude "Extrusion1" add sketch "Sketch1" along normal blind 2 contours A9 A15 L34 L33 L32 A16 A42 A30 A35 A31 A43 A17 L35 L36 L37 A18 A12 A21 L38 L39 L40 A19 A46 A32 A34 A33 A47 A14 L41 L42 L43 A13 A11 A110 A23 L44 L45 L46 A22 A45 A37 A36 A38 A44 A25 L49 L48 L47 A24 A10 A27 L50 L51 L52 A26 A49 A39 A40 A41 A48 A28 L53 L54 L55 A29
body "Solid1"
